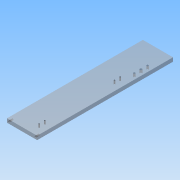
# Autodesk Inventor part: Tunel_SidePanel2
Saved by Autodesk Inventor 2016 (Build 200138000, 138)
## iProperties
Created: 2014-10-15
Part Number: Tunel_SidePanel2
Material: Polycarbonat, klar
Document SubType Name: Modeling
Designer: Gero Hofmann
Density: 1.2 g/cm^3
Appearance: Polycarbonat - klar
Author: Gero Hofmann
Autodesk Inventor part; units mm, degrees
ref_plane "YZ Plane" through (0, 0, 0) normal (1, 0, 0) x (0, 1, 0)
ref_plane "XZ Plane" through (0, 0, 0) normal (0, 1, 0) x (-1, 0, 0)
ref_plane "XY Plane" through (0, 0, 0) normal (0, 0, 1) x (1, 0, 0)
sketch "Skizze1" plane through (0, 0, 0) normal (0, 0, 1) x (1, 0, 0)
  line L0 (40, 180) -> (-40, 180)
  line L1 (-40, 180) -> (-40, -180)
  line L2 (-40, -180) -> (40, -180)
  line L3 (40, -180) -> (40, 180)
  line L4 (40, 180) -> (-40, -180) construction
  line L5 (-40, 180) -> (40, -180) construction
  point P0 (0, 0)
  dimension "d0" = 80
  dimension "d1" = 360
  constraints: 12 end point, 2 midpoint, 2 parallel, 1 horizontal, 1 perpendicular
  measures "d0" distance of L1.end L2.end
  measures "d1" distance of L0.end L1.end
extrude "Extrusion1" add sketch "Skizze1" along normal blind 10
sketch "Skizze2" plane through (0, 0, 10) normal (0, 0, 1) x (1, 0, 0)
  line L0 (40, 180) -> (-40, 180) projected
  line L1 (40, -180) -> (40, 180) projected
  point P0 (0, 0)
  point P1 (25, 110)
  dimension "d16" = 15
  dimension "d17" = 70
  measures "d16" distance from line of L1 point (25, 110)
  measures "d17" distance from line of point (25, 110) L0
hole "Bohrung2" at (25, 110, 10) direction (0, 0, -1) diameter 6 end through all
sketch "Skizze4" plane through (0, 0, 0) normal (0, 0, -1) x (-1, 0, 0)
  line L0 (40, -180) -> (-40, -180) projected
  line L1 (40, 180) -> (40, -180) projected
  line L2 (-15, -150) -> (-15, -135) construction
  point P0 (0, 0)
  dimension "d34" = 15
  dimension "d35" = 30
  dimension "d36" = 55
  constraints: 2 end point, 1 parallel
  measures "d34" distance of L2.start L2.end
  measures "d35" distance from line of L0 L2.start
  measures "d36" distance between parallel lines of L1 L2
hole "Bohrung4" at (15, -150, 0) at (15, -135, 0) direction (0, 0, 1) diameter 3.242 end through all thread size "M4x0.7" class "6H" standard "ISO Metric profile"
pattern_linear "Rechteckige Anordnung2" count 2 spacing 200 along (0, 1, 0) of "Bohrung4"
sketch "Skizze5" plane through (-40, -180, 0) normal (0, -1, 0) x (1, 0, 0)
  line L0 (0, 0) -> (80, 0) projected
  line L1 (0, 0) -> (0, 10) projected
  line L2 (5, 5) -> (75, 5)
  point P0 (40, 0)
  point P1 (40, 5)
  point P2 (40, 0)
  point P3 (0, 5)
  dimension "d47" = 5
  constraints: 3 midpoint, 2 end point, 1 perpendicular, 1 point on line, 1 vertical alignment
  measures "d47" distance from line of L1 L2.start
hole "Bohrung5" at (-35, -180, 5) at (35, -180, 5) direction (0, 1, 0) diameter 4.134 depth 10 tip angle 118 thread size "M5x0.8" class "6H" standard "ISO Metric profile"
sketch "Skizze6" plane through (0, 0, 0) normal (0, 0, -1) x (-1, 0, 0)
  circle A0 centre (-25, 110) radius 3 projected
  line L0 (40, 180) -> (40, -180) projected
  line L1 (-25, 127.5) -> (-25, 92.5)
  point P0 (0, 0)
  dimension "d55" = 35
  constraints: 2 end point, 1 coincident, 1 midpoint, 1 parallel
  measures "d55" distance of L1.start L1.end
hole "Bohrung6" at (25, 127.5, 0) at (25, 92.5, 0) direction (0, 0, 1) diameter 5 end through all
